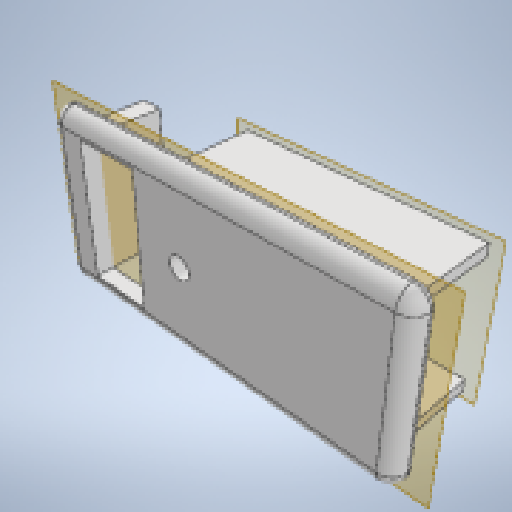
# Autodesk Inventor part: rf_tester_top
Saved by Autodesk Inventor 2025 (Build 290162000, 162)
## iProperties
Created: 2025-01-11
Part Number: rf_tester_top
Material: Generic
Document SubType Name: Modeling
Designer: Jacob
Density: 1 g/cm^3
Appearance: Default
Author: Jacob
Autodesk Inventor part; units mm, degrees
ref_plane "YZ Plane" through (0, 0, 0) normal (1, 0, 0) x (0, 1, 0)
ref_plane "XZ Plane" through (0, 0, 0) normal (0, 1, 0) x (-1, 0, 0)
ref_plane "Work Plane1" through (0, 0, 0) normal (0, 0, 1) x (1, 0, 0)
sketch "Sketch1" plane through (0, 0, 0) normal (0, 0, 1) x (1, 0, 0)
  arc A0 (-22.65, 11.4) -> (-24.65, 9.4) centre (-22.65, 9.4) ccw projected
  line L0 (-24.65, 9.4) -> (-24.65, -9.4) projected
  arc A1 (-24.65, -9.4) -> (-22.65, -11.4) centre (-22.65, -9.4) ccw projected
  line L1 (-22.65, -11.4) -> (22.65, -11.4) projected
  arc A2 (22.65, -11.4) -> (24.65, -9.4) centre (22.65, -9.4) ccw projected
  line L2 (24.65, -9.4) -> (24.65, 9.4) projected
  arc A3 (24.65, 9.4) -> (22.65, 11.4) centre (22.65, 9.4) ccw projected
  line L3 (22.65, 11.4) -> (-22.65, 11.4) projected
  line L4 (22.25, 9) -> (22.25, -9) projected
  line L5 (22.25, -9) -> (-8.35, -9) projected
  line L6 (-8.35, -2.5) -> (-8.35, -9) projected
  line L7 (-10.6, -2.5) -> (-8.35, -2.5) projected
  line L8 (-10.6, -9) -> (-10.6, -2.5) projected
  line L9 (-10.6, -9) -> (-22.25, -9) projected
  line L10 (-22.25, -9) -> (-22.25, 9) projected
  line L11 (-22.25, 9) -> (-10.6, 9) projected
  line L12 (-10.6, 2.5) -> (-10.6, 9) projected
  line L13 (-8.35, 2.5) -> (-10.6, 2.5) projected
  line L14 (-8.35, 9) -> (-8.35, 2.5) projected
  line L15 (-8.35, 9) -> (22.25, 9) projected
  line L16 (-20.5, -9) -> (-20.5, -4.5) projected
  line L17 (-20.5, 4.5) -> (-20.5, 9) projected
  line L18 (-20.5, -4.5) -> (-20.5, 4.5)
  line L19 (-10.6, -2.5) -> (-10.6, 2.5)
  line L20 (22.25, -7.5) -> (-8.35, -7.5)
  line L21 (-8.35, 7.5) -> (22.25, 7.5)
  point P0 (0, 0)
  dimension "d0" = 1.5
  dimension "d1" = 1.5
  constraints: 8 end point, 4 point on line, 2 perpendicular, 1 collinear, 1 vertical
  measures "d0" distance between parallel lines of L5 L20
  measures "d1" distance between parallel lines of L15 L21
ref_plane "Work Plane2" through (0, 0, -11.8) normal (0, 0, 1) x (1, 0, 0)
extrude "Extrusion1" add sketch "Sketch1" against normal up to surface (11.8 mm away) contours L4 L21 L14 L15 | L4 L5 L6 L20
ref_plane "Work Plane3" through (0, 0, 0) normal (0, 0, 1) x (1, 0, 0)
sketch "Sketch2" plane through (0, 0, 0) normal (0, 0, 1) x (1, 0, 0)
  line L0 (-22.25, -9) -> (-22.25, 9) projected
  line L1 (-10.6, -9) -> (-10.6, -2.5) projected
  line L2 (-10.6, 2.5) -> (-10.6, 9) projected
  line L3 (-10.6, -2.5) -> (-10.6, 2.5)
  line L4 (-10.6, -8.875) -> (-19.35, -8.875)
  line L5 (-19.35, -8.875) -> (-19.35, 8.875)
  line L6 (-19.35, 8.875) -> (-10.6, 8.875)
  line L7 (-10.6, 8.875) -> (-10.6, -8.875)
  line L8 (-19.35, -8.875) -> (-22.25, -8.875)
  line L9 (-19.35, 8.875) -> (-22.25, 8.875)
  point P0 (0, 0)
  point P1 (-10.6, 0)
  dimension "d4" = 17.75
  dimension "d5" = 8.75
  constraints: 14 end point, 2 horizontal, 2 midpoint, 2 parallel, 2 perpendicular, 2 point on line, 1 vertical
  measures "d4" distance of L4.end L5.end
  measures "d5" distance of L4.start L4.end
ref_plane "Work Plane4" through (-22.25, -9, -8.6) normal (0, 0, 1) x (1, 0, 0)
extrude "Extrusion2" add sketch "Sketch2" against normal up to surface (8.6 mm away) contours L0 L9 L5 L8
sketch "Sketch3" plane through (0, 0, 0) normal (0, 0, 1) x (1, 0, 0)
  arc A0 (-22.65, 11.4) -> (-24.65, 9.4) centre (-22.65, 9.4) ccw projected
  line L0 (-24.65, 9.4) -> (-24.65, -9.4) projected
  arc A1 (-24.65, -9.4) -> (-22.65, -11.4) centre (-22.65, -9.4) ccw projected
  line L1 (-22.65, -11.4) -> (22.65, -11.4) projected
  arc A2 (22.65, -11.4) -> (24.65, -9.4) centre (22.65, -9.4) ccw projected
  line L2 (24.65, -9.4) -> (24.65, 9.4) projected
  arc A3 (24.65, 9.4) -> (22.65, 11.4) centre (22.65, 9.4) ccw projected
  line L3 (22.65, 11.4) -> (-22.65, 11.4) projected
  line L4 (22.25, 9) -> (22.25, -9) projected
  line L5 (22.25, -9) -> (-8.35, -9) projected
  line L6 (-8.35, -2.5) -> (-8.35, -9) projected
  line L7 (-10.6, -2.5) -> (-8.35, -2.5) projected
  line L8 (-10.6, -9) -> (-10.6, -2.5) projected
  line L9 (-10.6, -9) -> (-22.25, -9) projected
  line L10 (-22.25, -9) -> (-22.25, 9) projected
  line L11 (-22.25, 9) -> (-10.6, 9) projected
  line L12 (-10.6, 2.5) -> (-10.6, 9) projected
  line L13 (-8.35, 2.5) -> (-10.6, 2.5) projected
  line L14 (-8.35, 9) -> (-8.35, 2.5) projected
  line L15 (-8.35, 9) -> (22.25, 9) projected
  line L16 (-19.35, -8.875) -> (-19.35, 8.875) projected
  line L17 (-19.35, -9) -> (-10.6, -9)
  line L18 (-10.6, -9) -> (-10.6, 9)
  line L19 (-10.6, 9) -> (-19.35, 9)
  line L20 (-19.35, 9) -> (-19.35, -9)
  point P0 (0, 0)
  point P1 (-19.35, 0)
  constraints: 8 end point, 2 midpoint, 2 parallel, 1 horizontal, 1 perpendicular
extrude "Extrusion3" add sketch "Sketch3" along normal blind 2.4 contours L3 A3 L2 A2 L1 A1 L0 A0 | L4 L5 L6 L7 L18 L13 L14 L15 | L20 L16 L9 L10 L11
fillet "Fillet1" radius 2 8 edges at (-24.0642, 10.8142, 2.4) (-24.65, 0, 2.4) (-24.0642, -10.8142, 2.4) (0, -11.4, 2.4) (24.0642, -10.8142, 2.4) (24.65, 0, 2.4) (24.0642, 10.8142, 2.4) (0, 11.4, 2.4)
sketch "Sketch4" plane through (0, 0, 2.4) normal (0, 0, 1) x (1, 0, 0)
  line L0 (22.25, 9) -> (22.25, -9) projected
  line L1 (22.25, -9) -> (-8.35, -9) projected
  line L2 (-8.35, -2.5) -> (-8.35, -9) projected
  circle A0 centre (-4.05, 0) radius 1.5
  line L3 (22.25, 0) -> (28.5402, 0) construction
  point P0 (0, 0)
  dimension "d11" = 3
  dimension "d12" = 4.3
  constraints: 2 end point, 1 centre point, 1 horizontal, 1 midpoint, 1 point on line
  measures "d11" diameter of A0
  measures "d12" distance from line of L2 A0.centre
extrude "Extrusion4" cut sketch "Sketch4" against normal up to surface (2.4 mm away)
equation "\"d1\" = d0"
body "Solid1"
